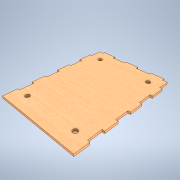
# Autodesk Inventor part: TableBottom
Saved by Autodesk Inventor 2021 (Build 250183000, 183)
## iProperties
Created: 2021-03-11
Part Number: TableBottom
Material: Wood (Cherry)
Document SubType Name: Modeling
Designer: ZiweZhang
Density: 0.63 g/cm^3
Appearance: Cherry - Natural Low Gloss
Author: ZiweZhang
Autodesk Inventor part; units mm, degrees
ref_plane "YZ Plane" through (0, 0, 0) normal (1, 0, 0) x (0, 1, 0)
ref_plane "XZ Plane" through (0, 0, 0) normal (0, 1, 0) x (-1, 0, 0)
ref_plane "XY Plane" through (0, 0, 0) normal (0, 0, 1) x (1, 0, 0)
sketch "Sketch2" plane through (0, 0, 0) normal (0, 1, 0) x (-1, 0, 0)
  line L0 (0, 0) -> (105, 0)
  line L1 (105, 0) -> (105, -140)
  line L2 (105, -140) -> (0, -140)
  line L3 (0, -140) -> (0, 0)
  point P0 (75, -100)
  dimension "d4" = 105
  dimension "d5" = 140
  constraints: 8 end point, 2 parallel, 1 horizontal, 1 perpendicular
  measures "d4" distance of L1.end L2.end
  measures "d5" distance of L0.end L1.end
extrude "Extrusion2" add sketch "Sketch2" along normal blind 3
sketch "Sketch3" plane through (0, 0, 0) normal (0, -1, 0) x (1, 0, 0)
  line L0 (-105, 0) -> (0, 0) projected
  line L1 (-105, -140) -> (-105, 0) projected
  line L2 (0, -17.5) -> (-3, -17.5)
  line L3 (-3, -17.5) -> (-3, -35)
  line L4 (-3, -35) -> (0, -35)
  line L5 (0, -35) -> (0, -52.5)
  line L6 (0, -52.5) -> (-3, -52.5)
  line L7 (-3, -52.5) -> (-3, -70)
  line L8 (-3, -70) -> (0, -70)
  line L9 (0, -70) -> (0, -87.5)
  line L10 (0, -87.5) -> (-3, -87.5)
  line L11 (-3, -87.5) -> (-3, -105)
  line L12 (-3, -105) -> (0, -105)
  line L13 (0, -105) -> (0, -122.5)
  line L14 (0, -122.5) -> (-3, -122.5)
  line L15 (-3, -122.5) -> (-3, -140)
  line L16 (0, -17.5) -> (0, 0)
  line L17 (-105, 0) -> (0, 0) projected
  line L18 (-105, -140) -> (-105, 0) projected
  line L19 (0, 0) -> (-105, 0)
  line L20 (-105, 0) -> (-105, -17.5)
  line L21 (-105, -17.5) -> (-102, -17.5)
  line L22 (-102, -17.5) -> (-102, -35)
  line L23 (-102, -35) -> (-105, -35)
  line L24 (-105, -35) -> (-105, -52.5)
  line L25 (-102, -52.5) -> (-105, -52.5)
  line L26 (-102, -52.5) -> (-102, -70)
  line L27 (-102, -70) -> (-105, -70)
  line L28 (-105, -70) -> (-105, -87.5)
  line L29 (-105, -87.5) -> (-102, -87.5)
  line L30 (-102, -87.5) -> (-102, -105)
  line L31 (-102, -105) -> (-105, -105)
  line L32 (-105, -105) -> (-105, -122.5)
  line L33 (-105, -122.5) -> (-102, -122.5)
  line L34 (-102, -122.5) -> (-102, -137)
  line L35 (0, -140) -> (-105, -140) projected
  line L36 (-105, -122.5) -> (-105, -105)
  line L37 (-102, -137) -> (-96.25, -137)
  line L38 (-96.25, -137) -> (-96.25, -140)
  line L39 (-96.25, -140) -> (-78.75, -140)
  line L40 (-52.5, -140) -> (-35, -140)
  line L41 (-17.5, -140) -> (-3, -140)
  line L42 (-3, -140) -> (-3, -137)
  line L43 (-61.25, -140) -> (-43.75, -140)
  line L44 (-43.75, -140) -> (-43.75, -137)
  line L45 (-43.75, -137) -> (-26.25, -137)
  line L46 (-26.25, -137) -> (-26.25, -140)
  line L47 (-26.25, -140) -> (-8.75, -140)
  line L48 (-8.75, -140) -> (-8.75, -137)
  line L49 (-8.75, -137) -> (-3, -137)
  line L50 (-96.25, -137) -> (-96.25, -140)
  line L51 (-96.25, -140) -> (-78.75, -140)
  line L52 (-78.75, -140) -> (-78.75, -137)
  line L53 (-78.75, -137) -> (-61.25, -137)
  line L54 (-61.25, -137) -> (-61.25, -140)
  line L55 (-61.25, -140) -> (-43.75, -140)
  line L56 (-26.25, -140) -> (-8.75, -140)
  point P0 (-17.5, -137)
  dimension "d51" = 3
  dimension "d52" = 17.5
  dimension "d53" = 17.5
  dimension "d54" = 17.5
  dimension "d55" = 17.5
  dimension "d56" = 17.5
  dimension "d58" = 3
  dimension "d65" = 17.5
  dimension "d66" = 17.5
  dimension "d67" = 17.5
  dimension "d69" = 5.75
  dimension "d70" = 5.75
  dimension "d71" = 17.5
  constraints: 104 end point, 19 point on line, 17 perpendicular, 6 horizontal, 2 vertical, 1 collinear, 1 midpoint, 8 other
  measures "d51" distance of L2.start L2.end
  measures "d52" distance of L2.end L3.end
  measures "d53" distance of L4.end L5.end
  measures "d54" distance of L8.end L9.end
  measures "d55" distance of L10.end L11.end
  measures "d56" distance of L12.end L13.end
  measures "d58" distance of L20.end L21.end
  measures "d65" distance of L43.start L43.end
  measures "d66" distance of L44.end L45.end
  measures "d67" distance of L46.end L47.end
  measures "d69" distance of L34.end L37.end
  measures "d70" distance of L48.end L42.end
  measures "d71" distance of L38.end L39.end
extrude "Extrusion3" cut sketch "Sketch3" against normal blind 3 contours L0 L16 L2 L3 L4 L5 L6 L7 L8 L9 L10 L11 L12 L13 L14 L15 L49 L48 L35 L46 L45 L44 L54 L53 L52 L38 L37 L34 L33 L1 L31 L30 L29 L27 L26 L25 L23 L22 L21 keep common part
sketch "Sketch5" plane through (0, 3, 0) normal (0, 1, 0) x (1, 0, 0)
  circle A0 centre (-27.25, 36) radius 3
  line L0 (0, 0) -> (0, 17.5) projected
  line L1 (0, 0) -> (0, 17.5)
  line L2 (-105, 0) -> (0, 0) projected
  line L3 (0, 0) -> (-17.5, 0)
  circle A1 centre (-77.75, 36) radius 3
  circle A2 centre (-27.25, 104) radius 3
  circle A3 centre (-77.75, 104) radius 3
  line L4 (-3, 122.5) -> (-3, 137) projected
  line L5 (-26.25, 137) -> (-43.75, 137) projected
  line L6 (0, 105) -> (0, 122.5) projected
  line L7 (-8.75, 140) -> (-26.25, 140) projected
  dimension "d72" = 17.5
  dimension "d75" = 50.5
  dimension "d78" = 68
  dimension "d81" = 6
  dimension "d84" = 27.25
  dimension "d85" = 36
  constraints: 4 centre point, 4 end point, 1 coincident, 1 collinear, 1 horizontal, 1 point on line, 1 vertical, 6 other
  measures "d72" distance of L0.start L3.end
  measures "d75" distance of A0.centre A1.centre
  measures "d78" distance of A0.centre A2.centre
  measures "d81" diameter of A0
  measures "d84" distance from line of A2.centre L6
  measures "d85" distance from line of A2.centre L7
extrude "Extrusion4" cut sketch "Sketch5" against normal blind 2.5
body "Solid2"
